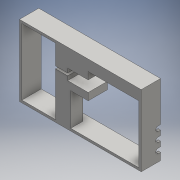
# Autodesk Inventor part: Lag4
Saved by Autodesk Inventor 2016 (Build 200138000, 138)
## iProperties
Created: 2016-12-12
Part Number: Lag4
Material: Generic
Document SubType Name: Modeling
Designer: Simon
Density: 1 g/cm^3
Appearance: Default
Author: Simon
Autodesk Inventor part; units mm, degrees
ref_plane "YZ Plane" through (0, 0, 0) normal (1, 0, 0) x (0, 1, 0)
ref_plane "XZ Plane" through (0, 0, 0) normal (0, 1, 0) x (-1, 0, 0)
ref_plane "XY Plane" through (0, 0, 0) normal (0, 0, 1) x (1, 0, 0)
sketch "Sketch1" plane through (0, 0, 0) normal (0, 1, 0) x (-1, 0, 0)
  line L0 (-58.5, 29.5) -> (42.5, 29.5)
  line L1 (42.5, 29.5) -> (42.5, -29.5)
  line L2 (42.5, -29.5) -> (-58.5, -29.5)
  line L3 (-58.5, -29.5) -> (-58.5, 29.5)
  line L4 (0, 10) -> (2.5, 10)
  line L5 (2.5, 10) -> (12.5, 10)
  line L6 (-14.5, 20.5) -> (-56.5, 20.5)
  line L7 (-56.5, 20.5) -> (-56.5, -0.5)
  line L8 (-56.5, -0.5) -> (-14.5, -0.5)
  line L9 (-14.5, -0.5) -> (-14.5, 20.5)
  line L10 (12.5, 11) -> (12.5, 9)
  line L11 (12.5, 9) -> (2.5, 9)
  line L12 (12.5, 11) -> (2.5, 11)
  line L13 (40.5, 27.5) -> (12.5, 27.5)
  line L14 (12.5, 27.5) -> (12.5, -27.5)
  line L15 (12.5, -27.5) -> (40.5, -27.5)
  line L16 (40.5, -27.5) -> (40.5, 27.5)
  line L17 (12.5, 27.5) -> (12.5, 29.5)
  line L18 (12.5, -27.5) -> (12.5, -29.5)
  line L19 (0, 0) -> (0, 10)
  line L20 (2.5, 11) -> (2.5, 9)
  line L21 (2.5, 14.5) -> (2.5, 5.5)
  line L22 (2.5, 5.5) -> (-14.5, 5.5)
  line L23 (2.5, 14.5) -> (-14.5, 14.5)
  line L24 (12.5, 0) -> (0, 0)
  line L25 (-56.5, -0.5) -> (12.5, -0.5)
  line L26 (12.5, -0.5) -> (12.5, -27.5)
  line L27 (12.5, -27.5) -> (-56.5, -27.5)
  line L28 (-56.5, -27.5) -> (-56.5, -0.5)
  line L29 (2.5, 5.5) -> (2.5, 0)
  point P0 (-8, 29.5)
  point P1 (0, 5.5)
  dimension "d2" = 2.5
  dimension "d3" = 10
  dimension "d4" = 2
  dimension "d5" = 21
  dimension "d6" = 42
  dimension "d9" = 28
  dimension "d10" = 55
  dimension "d13" = 10
  dimension "d14" = 9
  dimension "d15" = 17
  dimension "d16" = 2
  dimension "d17" = 2
  dimension "d20" = 2
  dimension "d28" = 101
  dimension "d29" = 59
  dimension "d34" = 42
  dimension "d35" = 27
  dimension "d37" = 12.5
  constraints: 60 end point, 11 perpendicular, 8 parallel, 7 horizontal, 7 point on line, 5 midpoint, 4 vertical, 2 collinear
  measures "d2" distance of L4.end L4.start
  measures "d3" distance of L4.end L5.end
  measures "d4" distance of L10.start L10.end
  measures "d5" distance of L8.end L6.start
  measures "d6" distance of L6.start L6.end
  measures "d9" distance of L14.end L15.end
  measures "d10" distance of L15.end L13.start
  measures "d13" distance from line of L19.start L5
  measures "d14" distance of L21.start L21.end
  measures "d15" distance of L21.start L23.end
  measures "d16" distance between parallel lines of L1 L16
  measures "d17" distance between parallel lines of L0 L13
  measures "d20" distance between parallel lines of L7 L3
  measures "d28" distance between parallel lines of L3 L1
  measures "d29" distance between parallel lines of L0 L2
  measures "d34" distance between parallel lines of L9 L28
  measures "d35" distance between parallel lines of L27 L25
  measures "d37" distance between parallel lines of L14 L19
sketch "Sketch2" plane through (0, 0, 0) normal (0, 1, 0) x (-1, 0, 0)
  line L0 (0, 0) -> (12.5, 0) projected
  line L1 (40.5, -27.5) -> (-56.5, -27.5) projected
  line L2 (12.5, 0) -> (12.5, -27.5)
  line L3 (12.5, 0) -> (0, 0)
  line L4 (0, 0) -> (0, -27.5)
  line L5 (0, -27.5) -> (12.5, -27.5)
  line L6 (12.5, -27.5) -> (12.5, 0)
  dimension "d36" = 56.5
  constraints: 10 end point, 3 point on line, 2 parallel, 2 perpendicular, 1 horizontal
  measures "d36" distance from line of L1.end L4
extrude "Extrusion5" add sketch "Sketch2" along normal blind 10
extrude "Extrusion6" add sketch "Sketch1" along normal blind 16 contours L0 L17 L14 L12 L21 L23 L9 L6 L7 L28 L27 L18 L2 L3 | L0 L1 L2 L18 L15 L16 L13 L17 | L25 L9 L22 L19 L24 L14 | L14 L24 L29 L21 L11 | L24 L19 L22 L29
sketch "Sketch3" plane through (0, 16, 0) normal (0, 1, 0) x (1, 0, 0)
  line L0 (56.5, 3.5) -> (56.5, 7.5)
  line L1 (56.5, 7.5) -> (56.5, 11.5)
  line L2 (56.5, 11.5) -> (56.5, 15.5)
  line L3 (56.5, 15.5) -> (56.5, 19.5)
  line L4 (56.5, 19.5) -> (56.5, 23.5)
  line L5 (56.5, 23.5) -> (56.5, 27.5)
  line L6 (58.5, -29.5) -> (58.5, 29.5) projected
  line L7 (56.5, 23.5) -> (58.5, 23.5)
  line L8 (58.5, -29.5) -> (58.5, 29.5) projected
  line L9 (56.5, 19.5) -> (58.5, 19.5)
  line L10 (56.5, 15.5) -> (58.5, 15.5)
  line L11 (56.5, 11.5) -> (58.5, 11.5)
  line L12 (56.5, 7.5) -> (58.5, 7.5)
  line L13 (56.5, 3.5) -> (58.5, 3.5)
  point P0 (0, 0)
  dimension "d30" = 4
  constraints: 24 end point, 10 point on line, 5 collinear, 4 parallel, 2 perpendicular, 2 vertical, 1 coincident
  measures "d30" distance of L4.end L5.end
extrude "Extrusion7" cut sketch "Sketch3" against normal blind 4 contours L0 L12 L6 L13 | L2 L10 L6 L11 | L4 L7 L6 L9
fillet "Fillet1" radius 2 6 edges at (57.5, 12, -3.5) (57.5, 12, -11.5) (57.5, 12, -19.5) (57.5, 12, -23.5) (57.5, 12, -15.5) (57.5, 12, -7.5)
body "Solid4"
